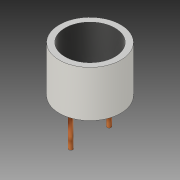
# Autodesk Inventor part: transducer
Saved by Autodesk Inventor 2019 (Build 230136000, 136)
## iProperties
Created: 2019-01-04
Part Number: transducer
Material: Generic
Document SubType Name: Modeling
Designer: Callum Snowden
Mass: 1.10034 g
Surface Area: 14.7341 cm^2
Volume: 1.10034 cm^3
Density: 1 g/cm^3
Appearance: Default
Author: Callum Snowden
Autodesk Inventor part; units mm, degrees
ref_plane "YZ Plane" through (0, 0, 0) normal (1, 0, 0) x (0, 1, 0)
ref_plane "XZ Plane" through (0, 0, 0) normal (0, 1, 0) x (-1, 0, 0)
ref_plane "XY Plane" through (0, 0, 0) normal (0, 0, 1) x (1, 0, 0)
sketch "Sketch1" plane through (0, 0, 0) normal (0, 1, 0) x (-1, 0, 0)
  line L0 (0, -11.2) -> (0, 11.2) construction
  line L1 (-11.2, 0) -> (11.2, 0) construction
  circle A0 centre (0, 0) radius 8
  dimension "d0" = 16
  constraints: 1 centre point, 1 coincident
  measures "d0" diameter of A0
extrude "Extrusion1" add sketch "Sketch1" along normal blind 12
sketch "Sketch2" plane through (0, 12, 0) normal (0, 1, 0) x (1, 0, 0)
  circle A0 centre (0, 0) radius 6.5
  dimension "d3" = 13
  constraints: 1 centre point, 1 coincident
  measures "d3" diameter of A0
extrude "Extrusion2" cut sketch "Sketch2" against normal blind 10
sketch "Sketch4" plane through (0, 0, 0) normal (0, -1, 0) x (1, 0, 0)
  line L0 (0, 11.2) -> (0, -11.2) construction
  line L1 (-11.2, 0) -> (11.2, 0) construction
  circle A0 centre (0, 5) radius 0.5
  circle A1 centre (0, -5) radius 0.5
  point P0 (0, 0)
  dimension "d39" = 1
  dimension "d40" = 1
  dimension "d41" = 10
  constraints: 2 centre point, 2 point on line, 1 symmetric about line
  measures "d39" diameter of A0
  measures "d40" diameter of A1
  measures "d41" distance of A1.centre A0.centre
extrude "Extrusion4" add sketch "Sketch4" along normal blind 9.5
equation "\"d40\" = d39"
body "Solid1"
